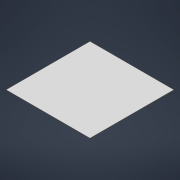
# Autodesk Inventor part: floor
Saved by Autodesk Inventor 2022 (Build 260153000, 153)
## iProperties
Created: 2022-02-06
Part Number: floor
Material: 一般
Document SubType Name: Modeling
Designer: shiokaze
Density: 1 g/cm^3
Appearance: 既定
Mass: 40 g
Surface Area: 808 cm^2
Volume: 40 cm^3
Author: shiokaze
Autodesk Inventor part; units mm, degrees
ref_plane "YZ Plane" through (0, 0, 0) normal (1, 0, 0) x (0, 1, 0)
ref_plane "XZ Plane" through (0, 0, 0) normal (0, 1, 0) x (-1, 0, 0)
ref_plane "XY Plane" through (0, 0, 0) normal (0, 0, 1) x (1, 0, 0)
sketch "スケッチ1" plane through (0, 0, 0) normal (0, 1, 0) x (-1, 0, 0)
  line L0 (85.3868, 119.6275) -> (-114.6132, 119.6275)
  line L1 (-114.6132, 119.6275) -> (-114.6132, -80.3725)
  line L2 (-114.6132, -80.3725) -> (85.3868, -80.3725)
  line L3 (85.3868, -80.3725) -> (85.3868, 119.6275)
  point P0 (0, 0)
  dimension "d2" = 200
  dimension "d3" = 200
  constraints: 8 end point, 2 parallel, 1 horizontal, 1 perpendicular
  measures "d2" distance of L0.start L0.end
  measures "d3" distance of L2.end L0.start
extrude "押し出し1" add sketch "スケッチ1" along normal blind 1
